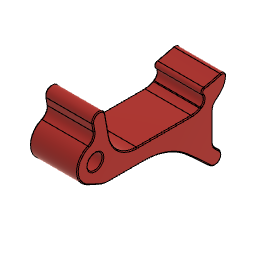
[a]_latch (Autodesk Fusion 360 design; units mm, degrees)
Autodesk Fusion 360 part; units mm, degrees
sketch "Sketch1" plane through (0, 0, 0) normal (1, 0, 0) x (0, 1, 0) in component "[a]_latch"
  spline S0 degree 3 poles (-10.6277, 6.4557) (-10.4802, 5.6222) (-10.1713, 4.8255) (-9.2656, 3.3954) (-8.6774, 2.7757) (-7.4408, 1.8988) (-6.8381, 1.5983) (-5.5622, 1.1918) (-4.8966, 1.0884) (-4.2271, 1.0884) knots 0 0 0 0 0.253919 0.253919 0.507838 0.507838 0.708696 0.708696 0.909554 0.909554 0.909554 0.909554
  line L0 (-10.6277, 6.4557) -> (-10.4802, 5.6222)
  line L1 (-10.4802, 5.6222) -> (-10.1713, 4.8255)
  line L2 (-10.1713, 4.8255) -> (-9.2656, 3.3954)
  line L3 (-9.2656, 3.3954) -> (-8.6774, 2.7757)
  line L4 (-8.6774, 2.7757) -> (-7.4408, 1.8988)
  line L5 (-7.4408, 1.8988) -> (-6.8381, 1.5983)
  line L6 (-6.8381, 1.5983) -> (-5.5622, 1.1918)
  line L7 (-5.5622, 1.1918) -> (-4.8966, 1.0884)
  line L8 (-4.8966, 1.0884) -> (-4.2271, 1.0884)
  line L9 (-10.6277, 6.4557) -> (-11.487, 11.3114)
  arc A0 (-11.487, 11.3114) -> (-14.4411, 10.7886) centre (-12.964, 11.05) ccw
  line L10 (-14.4411, 10.7886) -> (-14.1338, 9.0523)
  arc A1 (-15.3647, 6.8451) -> (-14.1338, 9.0523) centre (-16.1032, 8.7038) ccw
  arc A2 (-15.3647, 6.8451) -> (-15.5863, -0.7728) centre (-13.8325, 2.9884) ccw
  line L11 (-15.5863, -0.7728) -> (-12.862, -2.0432)
  arc A3 (-12.862, -2.0432) -> (-10.749, -2.5116) centre (-10.749, 2.4884) ccw
  line L12 (-10.749, -2.5116) -> (-2.5005, -2.5116)
  arc A4 (7.6148, -6.4355) -> (-2.5005, -2.5116) centre (-2.5005, -17.5116) ccw
  line L13 (7.6148, -6.4355) -> (12.7434, -11.1193)
  arc A5 (12.7434, -11.1193) -> (14.7665, -8.904) centre (13.7549, -10.0116) ccw
  line L14 (14.7665, -8.904) -> (13.9062, -8.1184)
  arc A6 (13.2549, -6.6416) -> (13.9062, -8.1184) centre (15.2549, -6.6416) ccw
  line L15 (13.2549, -6.6416) -> (13.2549, -0.2086)
  arc A7 (13.9874, 1.3385) -> (13.2549, -0.2086) centre (15.2549, -0.2086) ccw
  arc A8 (13.9874, 1.3385) -> (15.1677, 2.4015) centre (3.2133, 14.4884) ccw
  arc A9 (15.1677, 2.4015) -> (16.3522, 5.0986) centre (12.3549, 5.2455) ccw
  arc A10 (16.3522, 5.0986) -> (15.0788, 6.0971) centre (15.3529, 5.1354) ccw
  arc A11 (11.309, 5.2082) -> (15.0788, 6.0971) centre (3.5545, 46.5367) ccw
  arc A12 (11.309, 5.2082) -> (10.8832, 3.9768) centre (11.4473, 4.4711) ccw
  arc A13 (10.4966, 1.6845) -> (10.8832, 3.9768) centre (9.7549, 2.9884) ccw
  arc A14 (8.3883, 1.0884) -> (10.3175, 1.5843) centre (8.3883, 5.0884) ccw
  arc A15 (10.3175, 1.5843) -> (10.4966, 1.6845) centre (3.2133, 14.4884) ccw
  line L16 (8.3883, 1.0884) -> (-4.2271, 1.0884)
  circle A16 centre (-13.8325, 2.9884) radius 1.75
extrude "Extrude1" add sketch "Sketch1" along normal mid plane 11 in component "[a]_latch"
chamfer "Chamfer1" distance 0.2 angle 45 52 edges at (5.5, -11.0573, 8.8835) (5.5, -13.2254, 12.527) (5.5, -14.2874, 9.9204) (5.5, -14.3565, 7.7296) (5.5, -17.9807, 3.109) (5.5, -14.2242, -1.408) (5.5, -11.8312, -2.3931) (5.5, -6.6247, -2.5116) (5.5, 2.9244, -3.527) (5.5, 10.1791, -8.7774) (5.5, 14.8625, -11.0232) (5.5, 14.3363, -8.5112) (5.5, 13.425, -7.4486) (5.5, 13.2549, -3.4251) (5.5, 13.4473, 0.6473) (5.5, 14.59, 1.8562) (5.5, 16.0173, 3.6371) (5.5, 15.9699, 5.9223) (5.5, 13.2041, 5.6092) (5.5, 10.7385, 4.7162) (5.5, 11.234, 2.7389) (5.5, 10.4072, 1.6341) (5.5, 9.3843, 1.2143) (5.5, 2.0806, 1.0884) (5.5, -8.4061, 2.6098) (5.5, -15.464, 3.6212) (-5.5, -11.0573, 8.8835) (-5.5, -8.4061, 2.6098) (-5.5, 2.0806, 1.0884) (-5.5, 9.3843, 1.2143) (-5.5, 10.4072, 1.6341) (-5.5, 11.234, 2.7389) (-5.5, 10.7385, 4.7162) (-5.5, 13.2041, 5.6092) (-5.5, 15.9699, 5.9223) (-5.5, 16.0173, 3.6371) (-5.5, 14.59, 1.8562) (-5.5, 13.4473, 0.6473) (-5.5, 13.2549, -3.4251) (-5.5, 13.425, -7.4486) (-5.5, 14.3363, -8.5112) (-5.5, 14.8625, -11.0232) (-5.5, 10.1791, -8.7774) (-5.5, 2.9244, -3.527) (-5.5, -6.6247, -2.5116) (-5.5, -11.8312, -2.3931) (-5.5, -14.2242, -1.408) (-5.5, -17.9807, 3.109) (-5.5, -14.3565, 7.7296) (-5.5, -14.2874, 9.9204) (-5.5, -13.2254, 12.527) (-5.5, -15.464, 2.3555) in component "[a]_latch"
sketch "Sketch2" plane through (0, 13.2549, 0) normal (0, 1, 0) x (-1, 0, 0) in component "[a]_latch"
  line L0 (5.3, -6.6416) -> (5.3, -0.2086)
  line L1 (5.3, -0.2086) -> (-5.3, -0.2086)
  line L2 (-5.3, -0.2086) -> (-5.3, -6.6416)
  line L3 (-5.3, -6.6416) -> (5.3, -6.6416)
  line L4 (-1.7321, -1.9251) -> (1.7321, -1.9251)
  line L5 (1.7321, -1.9251) -> (0, -4.9251)
  line L6 (0, -4.9251) -> (-1.7321, -1.9251)
extrude "Extrude2" cut sketch "Sketch2" against normal blind 1 contours L4 L5 L6 in component "[a]_latch"
component "[a]_latch" placed x (1, 0, 0) y (0, 1, 0) z (0, 0, 1) at (0, 0, 0)
